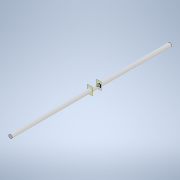
# Autodesk Inventor part: Держатель крыла
Saved by Autodesk Inventor 2022.1 (Build 261234000, 234)
## iProperties
Created: 2021-12-26
Part Number: Держатель крыла
Material: Типовые
Document SubType Name: Modeling
Designer: Grigori
Density: 1 g/cm^3
Appearance: По умолчанию
Author: Grigori
Autodesk Inventor part; units mm, degrees
ref_plane "YZ Plane" through (0, 0, 0) normal (1, 0, 0) x (0, 1, 0)
ref_plane "XZ Plane" through (0, 0, 0) normal (0, 1, 0) x (-1, 0, 0)
ref_plane "XY Plane" through (0, 0, 0) normal (0, 0, 1) x (1, 0, 0)
sketch "Эскиз1" plane through (0, 0, 0) normal (0, 0, 1) x (1, 0, 0)
  circle A0 centre (0, 0) radius 5
  dimension "d0" = 10
  constraints: 1 centre point, 1 coincident
  measures "d0" diameter of A0
extrude "Выдавливание1" add sketch "Эскиз1" along normal mid plane 450
ref_plane "РабПлоскость5" through (-6.4749, 10.717, -25) normal (0, 0, -1) x (1, 0, 0)
ref_plane "РабПлоскость4" through (-6.4749, 10.717, 0) normal (0, 0, -1) x (1, 0, 0)
sketch "Эскиз4" plane through (-6.4749, 10.717, -25) normal (0, 0, -1) x (1, 0, 0)
  circle A0 centre (6.4749, 10.717) radius 5
  dimension "d6" = 10
  constraints: 1 centre point, 1 coincident
  measures "d6" diameter of A0
